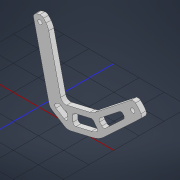
# Autodesk Inventor part: swing_arm_sm_x2
Saved by Autodesk Inventor 2022.2 (Build 262287010, 287A)
## iProperties
Created: 2022-03-19
Part Number: swing_arm_sm_x2
Material: Generisch
Document SubType Name: Modeling
Designer: sleib
Density: 1 g/cm^3
Appearance: Vorgabe
Author: sleib
Autodesk Inventor part; units mm, degrees
ref_plane "YZ Plane" through (0, 0, 0) normal (1, 0, 0) x (0, 1, 0)
ref_plane "XZ Plane" through (0, 0, 0) normal (0, 1, 0) x (-1, 0, 0)
ref_plane "XY Plane" through (0, 0, 0) normal (0, 0, 1) x (1, 0, 0)
sketch "Skizze1" plane through (6.6462, 35.3952, 4) normal (0, 0, 1) x (1, 0, 0)
  circle A0 centre (-1.4819, 27.5988) radius 1.7
  circle A1 centre (72.4299, 3.5807) radius 1.7
  line L0 (-6.5755, 28.4803) -> (5.7742, -25.0109)
  line L1 (7.9964, -28.1253) -> (18.1089, -34.4401)
  line L2 (5.4969, 25.0887) -> (14.9808, -15.9899)
  line L3 (19.7881, -18.9852) -> (38.2711, -14.6681)
  line L4 (70.7299, 9.8334) -> (42.2354, -12.7538)
  line L5 (49.4368, -26.2031) -> (78.3934, 0.9287)
  line L6 (22.5763, -35.1811) -> (40.4628, -31.0032)
  arc A2 (5.7742, -25.0109) -> (7.9964, -28.1253) centre (10.6431, -23.8868) ccw
  arc A3 (18.1089, -34.4401) -> (22.5763, -35.1811) centre (21.2342, -29.4352) ccw
  arc A4 (40.4628, -31.0032) -> (49.4368, -26.2031) centre (35.9895, -11.8514) ccw
  arc A5 (14.9808, -15.9899) -> (19.7881, -18.9852) centre (18.8783, -15.0901) ccw
  arc A6 (38.2711, -14.6681) -> (42.2354, -12.7538) centre (35.981, -4.8636) ccw
  arc A7 (74.5057, 9.794) -> (70.7299, 9.8334) centre (72.5935, 7.4824) ccw
  arc A8 (78.3934, 0.9287) -> (78.9159, 4.6593) centre (76.3421, 3.1179) ccw
  arc A9 (78.9159, 4.6593) -> (74.5057, 9.794) centre (61.7576, -5.6166) ccw
  arc A10 (-6.4652, 29.9708) -> (-6.5755, 28.4803) centre (-4.6703, 29.0887) ccw
  arc A11 (-5.4252, 31.4623) -> (-6.4652, 29.9708) centre (-1.0804, 27.3244) ccw
  arc A12 (-4.4188, 32.0336) -> (-5.4252, 31.4623) centre (-3.9769, 30.083) ccw
  arc A13 (1.3257, 31.6984) -> (-1.6126, 32.6692) centre (-0.9498, 29.7434) ccw
  arc A14 (5.4969, 25.0887) -> (3.3383, 29.3558) centre (-4.2468, 22.8392) ccw
  line L7 (-4.4188, 32.0336) -> (-1.6126, 32.6692)
  line L8 (1.3257, 31.6984) -> (3.3383, 29.3558)
  line L9 (13.7992, -20.5987) -> (8.256, -23.5195) construction
  line L10 (8.256, -23.5195) -> (21.1275, -31.5571) construction
  line L11 (21.1275, -31.5571) -> (20.3834, -24.2133) construction
  line L12 (20.3834, -24.2133) -> (13.7992, -20.5987) construction
  line L13 (24.3835, -21.8876) -> (40.478, -18.1284) construction
  line L14 (45.979, -25.6425) -> (24.9108, -30.5635) construction
  line L15 (24.9108, -30.5635) -> (24.3835, -21.8876) construction
  line L16 (44.6728, -15.8769) -> (63.3005, -1.111) construction
  line L17 (63.3005, -1.111) -> (66.4412, -4.7533) construction
  line L18 (66.4412, -4.7533) -> (49.0955, -21.0061) construction
  line L19 (49.0955, -21.0061) -> (44.6728, -15.8769) construction
  arc A15 (46.3062, -14.5821) -> (46.0339, -17.4555) centre (47.5486, -16.1494) ccw
  arc A16 (47.7343, -19.4275) -> (50.6165, -19.5809) centre (49.249, -18.1214) ccw
  arc A17 (65.0408, -6.0655) -> (65.188, -3.3) centre (63.6734, -4.606) ccw
  arc A18 (64.5537, -2.5643) -> (61.7967, -2.3031) centre (63.039, -3.8704) ccw
  line L20 (46.8841, -18.4415) -> (64.8709, -2.9322) construction
  arc A19 (11.335, -21.8971) -> (11.208, -25.3629) centre (12.2673, -23.6665) ccw
  arc A20 (17.6671, -29.3963) -> (20.7163, -27.4983) centre (18.7264, -27.6999) ccw
  arc A21 (15.248, -21.5115) -> (12.8475, -21.1002) centre (13.7798, -22.8696) ccw
  arc A22 (15.248, -21.5115) -> (18.8572, -23.4929) centre (20.0196, -17.0977) ccw
  arc A23 (20.4894, -25.2591) -> (18.8572, -23.4929) centre (18.4996, -25.4607) ccw
  arc A24 (26.0273, -21.5037) -> (24.4859, -23.5726) centre (26.4822, -23.4512) ccw
  arc A25 (41.2591, -19.1953) -> (39.1904, -18.4291) centre (39.6453, -20.3767) ccw
  arc A26 (24.767, -28.1983) -> (27.2183, -30.0245) centre (26.7634, -28.077) ccw
  line L21 (40.478, -18.1284) -> (45.979, -25.6425) construction
  arc A27 (39.5768, -27.1379) -> (43.2374, -25.7591) centre (36.165, -12.5311) ccw
  arc A28 (43.2374, -25.7591) -> (43.9082, -22.8139) centre (42.2944, -23.9954) ccw
  line L22 (46.3062, -14.5821) -> (61.7967, -2.3031)
  line L23 (64.5537, -2.5643) -> (65.188, -3.3)
  line L24 (65.0408, -6.0655) -> (50.6165, -19.5809)
  line L25 (47.7343, -19.4275) -> (46.0339, -17.4555)
  line L26 (41.2591, -19.1953) -> (43.9082, -22.8139)
  line L27 (39.1904, -18.4291) -> (26.0273, -21.5037)
  line L28 (24.767, -28.1983) -> (24.4859, -23.5726)
  line L29 (27.2183, -30.0245) -> (39.5768, -27.1379)
  line L30 (11.208, -25.3629) -> (17.6671, -29.3963)
  line L31 (20.7163, -27.4983) -> (20.4894, -25.2591)
  line L32 (12.8475, -21.1002) -> (11.335, -21.8971)
  point P0 (-6.6462, -35.3952)
  point P1 (43.2285, -21.8854)
  dimension "d0" = 3.4
  dimension "d1" = 3.4
  dimension "d2" = 11
  dimension "d3" = 3
  dimension "d6" = 3
  dimension "d7" = 20
  dimension "d8" = 2
  dimension "d9" = 3
  dimension "d10" = 6
  dimension "d11" = 2
  dimension "d12" = 10
  dimension "d13" = 4
  dimension "d14" = 2
  dimension "d15" = 2
  dimension "d16" = 2
  dimension "d17" = 2
  dimension "d18" = 23.75
  dimension "d19" = 2
  dimension "d20" = 2
  dimension "d21" = 2
  dimension "d22" = 2
  dimension "d23" = 68
  dimension "d24" = 2
  dimension "d25" = 2
  dimension "d26" = 2
  dimension "d29" = 2
  dimension "d30" = 15
  dimension "d31" = 6.5
  constraints: 66 end point, 54 point on circle, 49 tangent, 29 centre point, 24 point on line, 8 collinear, 7 parallel, 3 midpoint, 2 perpendicular, 25 other
  measures "d0" diameter of A0
  measures "d1" diameter of A1
  measures "d2" distance between parallel lines of L2 L0
  measures "d3" radius of A7
  measures "d6" radius of A8
  measures "d7" radius of A9
  measures "d8" radius of A10
  measures "d9" radius of A13
  measures "d10" radius of A11
  measures "d11" radius of A12
  measures "d12" radius of A14
  measures "d13" radius of A5
  measures "d14" radius of A18
  measures "d15" radius of A17
  measures "d16" radius of A16
  measures "d17" radius of A15
  measures "d18" distance between parallel lines of L17 L19
  measures "d19" radius of A19
  measures "d20" radius of A21
  measures "d21" radius of A23
  measures "d22" radius of A20
  measures "d23" angle of L11 L9
  measures "d24" radius of A24
  measures "d25" radius of A26
  measures "d26" radius of A25
  measures "d29" radius of A28
  measures "d30" radius of A27
  measures "d31" radius of A22
extrude "Extrusion1" add sketch "Skizze1" against normal blind 4
